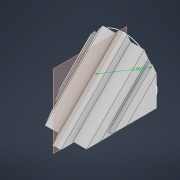
# Autodesk Inventor part: crossection rough
Saved by Autodesk Inventor 2022 (Build 260153000, 153)
## iProperties
Created: 2021-06-09
Part Number: crossection rough
Material: Generic
Document SubType Name: Modeling
Designer: sidsa
Density: 1 g/cm^3
Appearance: Default
Author: sidsa
## iProperties of the stored document crossection_3DPrint.ipt
Created: 2021-06-09
Part Number: crossection_3DPrint
Material: Generic
Document SubType Name: Modeling
Designer: sidsa
Density: 1 g/cm^3
Appearance: Default
Author: sidsa
Autodesk Inventor part; units mm, degrees
sketch "Sketch3" plane through (0, 0, 0) normal (0, 0, 1) x (1, 0, 0)
  circle A0 centre (0, 0) radius 25.4
  dimension "d5" = 50.8
  constraints: 1 centre point, 1 coincident
  measures "d5" diameter of A0
ref_plane "Work Plane1" through (12.7, 0, 0) normal (1, 0, 0) x (0, 1, 0)
ref_plane "Work Plane2" through (25.4, 0, 0) normal (1, 0, 0) x (0, 1, 0)
ref_plane "Work Plane4" through (-25.4, 0, 0) normal (1, 0, 0) x (0, 1, 0)
ref_plane "Work Plane3" through (-12.7, 0, 0) normal (1, 0, 0) x (0, 1, 0)
sketch "Sketch4" plane through (25.4, 0, 0) normal (1, 0, 0) x (0, 1, 0)
  line L0 (0, 0) -> (0, 0.0003)
  line L1 (0, 0) -> (0.0003, 0)
  line L2 (0.0003, 0) -> (0, 0.0003)
  dimension "d10" = 0.0003
  dimension "d11" = 0.0003
  constraints: 6 end point, 1 horizontal, 1 vertical
  measures "d10" distance of L0.start L0.end
  measures "d11" distance of L0.start L1.end
sketch "Sketch5" plane through (-25.4, 0, 0) normal (1, 0, 0) x (0, 1, 0)
  line L0 (0, 0) -> (0, 0.0003)
  line L1 (0, 0) -> (0.0003, 0)
  line L2 (0.0003, 0) -> (0, 0.0003)
  dimension "d12" = 0.0003
  dimension "d13" = 0.0003
  constraints: 6 end point, 1 horizontal, 1 vertical
  measures "d12" distance of L0.start L0.end
  measures "d13" distance of L0.start L1.end
ref_plane "Work Plane5" through (0, 0, 0) normal (1, 0, 0) x (0, 1, 0)
sketch "Sketch6" plane through (-12.7, 0, 0) normal (1, 0, 0) x (0, 1, 0)
  line L0 (0, 0) -> (21.997, 0)
  line L1 (0, 0) -> (-21.997, 0)
  line L2 (-21.997, 0) -> (-21.997, 43.9941)
  line L3 (-21.997, 43.9941) -> (21.997, 0)
  dimension "d15" = 21.9971
  dimension "d16" = 21.9971
  dimension "d17" = 43.9941
  constraints: 8 end point, 2 horizontal, 1 vertical
  measures "d15" distance of L0.start L0.end
  measures "d16" distance of L0.start L1.end
  measures "d17" distance of L1.end L2.end
sketch "Sketch7" plane through (12.7, 0, 0) normal (1, 0, 0) x (0, 1, 0)
  line L0 (0, 0) -> (21.997, 0)
  line L1 (0, 0) -> (-21.997, 0)
  line L2 (-21.997, 0) -> (-21.997, 43.9941)
  line L3 (-21.997, 43.9941) -> (21.997, 0)
  dimension "d18" = 21.9971
  dimension "d19" = 21.9971
  dimension "d20" = 43.9941
  constraints: 8 end point, 2 horizontal, 1 vertical
  measures "d18" distance of L0.start L0.end
  measures "d19" distance of L0.start L1.end
  measures "d20" distance of L1.end L2.end
sketch "Sketch8" plane through (0, 0, 0) normal (1, 0, 0) x (0, 1, 0)
  line L0 (0, 0) -> (25.4, 0)
  line L1 (0, 0) -> (-25.4, 0)
  line L2 (-25.4, 0) -> (-25.4, 50.8)
  line L3 (-25.4, 50.8) -> (25.4, 0)
  dimension "d21" = 25.4
  dimension "d22" = 25.4
  dimension "d23" = 50.8
  constraints: 8 end point, 2 horizontal, 1 perpendicular
  measures "d21" distance of L0.start L0.end
  measures "d22" distance of L0.start L1.end
  measures "d23" distance of L1.end L2.end
extrude "Extrusion2" add sketch "Sketch8" along normal mid plane 12.7
extrude "Extrusion3" add sketch "Sketch7" along normal mid plane 12.7
extrude "Extrusion4" add sketch "Sketch6" along normal mid plane 12.7
sketch "Sketch9" plane through (19.05, 0, 0) normal (1, 0, 0) x (0, 0, -1)
  line L0 (0, 0) -> (0, 15.24)
  line L1 (0, -21.997) -> (0, 21.997) projected
  line L2 (0, 0) -> (0, -15.24)
  line L3 (0, -15.24) -> (-30.48, -15.24)
  line L4 (-30.48, -15.24) -> (0, 15.24)
  dimension "d40" = 15.24
  dimension "d41" = 15.24
  dimension "d42" = 30.48
  constraints: 8 end point, 2 point on line, 1 perpendicular
  measures "d40" distance of L0.start L0.end
  measures "d41" distance of L0.start L2.end
  measures "d42" distance of L2.end L3.end
sketch "Sketch10" plane through (-19.05, 0, 0) normal (-1, 0, 0) x (0, 0, 1)
  line L0 (0, 0) -> (0, 15.24)
  line L1 (0, -21.997) -> (0, 21.997)
  line L2 (0, 0) -> (0, -15.24)
  line L3 (0, -15.24) -> (-30.48, -15.24)
  line L4 (-30.48, -15.24) -> (0, 15.24)
  line L5 (0, -15.24) -> (30.48, -15.24)
  line L6 (30.48, -15.24) -> (0, 15.24)
  dimension "d43" = 15.24
  dimension "d44" = 15.24
  dimension "d45" = 30.48
  constraints: 14 end point, 2 point on line, 1 perpendicular, 1 symmetric about line
  measures "d43" distance of L0.start L0.end
  measures "d44" distance of L0.start L2.end
  measures "d45" distance of L2.end L3.end
extrude "Extrusion5" add sketch "Sketch10" along normal blind 6.35 contours L0 L6 L5 L1
extrude "Extrusion6" add sketch "Sketch9" along normal blind 6.35
chamfer "Chamfer1" distance 3.175 angle 45 12 edges at (19.05, -21.997, 21.997) (25.4, -15.24, 15.24) (25.4, 0, 15.24) (19.05, 0, 21.997) (6.35, -25.4, 25.4) (6.35, 0, 25.4) (-6.35, 0, 25.4) (-6.35, -25.4, 25.4) (-19.05, 0, 21.997) (-19.05, -21.997, 21.997) (-25.4, 0, 15.24) (-25.4, -15.24, 15.24)
body "Solid3"
